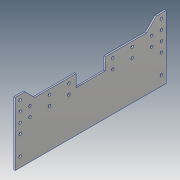
# Autodesk Inventor part: 200-40-BOGIE-CONNECTOR-06
Saved by Autodesk Inventor 2018.2 (Build 222227000, 227)
## iProperties
Manager: feesmrt
Company: FRANCOR
Part Number: 200-40-BOGIE-CONNECTOR-06
Project: Rescue Robot
Cost Center: -
Material: Aluminium 6061
Document SubType Name: Modeling
Designer: feesmrt
Engineer: feesmrt
Authority: feesmrt
Density: 2.7 g/cm^3
Appearance: Aluminium - flach
Description: Bogie Connector Verstärkungsplatte
Stock Number: 200-40-BOGIE-CONNECTOR-06
Mass: 165.052 g
Surface Area: 105.648 cm^2
Volume: 20.6315 cm^3
Subject: Rescue Robot
Author: feesmrt
Revision Number: 1
Title: Bogie Connector Verstärkungsplatte
Autodesk Inventor part; units mm, degrees
ref_plane "YZ Plane" through (0, 0, 0) normal (1, 0, 0) x (0, 1, 0)
ref_plane "XZ Plane" through (0, 0, 0) normal (0, 1, 0) x (-1, 0, 0)
ref_plane "XY Plane" through (0, 0, 0) normal (0, 0, 1) x (1, 0, 0)
sketch "Skizze1" plane through (0, 0, 0) normal (1, 0, 0) x (0, 1, 0)
  line L0 (-155, -65) -> (155, -65)
  line L1 (155, -65) -> (155, 65)
  line L2 (155, 65) -> (-155, 65)
  line L3 (-155, 65) -> (-155, -65)
  line L4 (-155, -65) -> (155, 65) construction
  line L5 (155, -65) -> (-155, 65) construction
  point P0 (0, 0)
  dimension "d43" = 310
  dimension "d44" = 130
  constraints: 12 end point, 2 midpoint, 2 parallel, 1 horizontal, 1 perpendicular
  measures "d43" distance of L1.end L2.end
  measures "d44" distance of L0.end L1.end
extrude "Grundlörper" add sketch "Skizze1" along normal blind 3
sketch "Skizze5" plane through (3, 0, 0) normal (1, 0, 0) x (0, 0, -1)
  line L0 (-65, -155) -> (65, -155) construction
  line L1 (-65, 155) -> (-65, -155) construction
  line L2 (65, 155) -> (-65, 155) construction
  line L3 (-147, 0) -> (147, 0) construction
  line L4 (0, -217) -> (0, 217) construction
  line L5 (-65, -135) -> (-45, -115)
  line L6 (-45, -115) -> (-45, -30)
  line L7 (-45, -30) -> (-20, -30)
  line L8 (-20, -30) -> (-20, 30)
  line L9 (-20, 30) -> (-45, 30)
  line L10 (-45, 30) -> (-45, 115)
  line L11 (-45, 115) -> (-65, 135)
  line L12 (-65, -135) -> (-65, 135)
  point P0 (0, 0)
  dimension "d47" = 20
  dimension "d48" = 20
  dimension "d49" = 20
  dimension "d50" = 60
  dimension "d51" = 25
  constraints: 16 end point, 3 perpendicular, 3 vertical, 2 point on line, 3 other
  measures "d47" distance from line of L0 L5.start
  measures "d48" horizontal distance of L5.start L5.end
  measures "d49" distance between parallel lines of L1 L6
  measures "d50" distance between parallel lines of L9 L7
  measures "d51" distance of L6.end L7.end
extrude "Aussschnitt" cut sketch "Skizze5" against normal through all
sketch "Skizze6" plane through (3, 0, 0) normal (1, 0, 0) x (0, 0, -1)
  line L0 (-65, -155) -> (65, -155) construction
  line L1 (-65, -135) -> (-65, -155) construction
  line L2 (-65, -145) -> (65, -145) construction
  line L3 (65, -155) -> (65, 155) construction
  line L4 (-35, -30) -> (-35, -155) construction
  line L5 (-45, -30) -> (-45, -115) construction
  line L6 (-15, 0) -> (-15, -155) construction
  line L7 (-147, 0) -> (147, 0) projected
  point P0 (-55, -145)
  point P1 (-35, -125)
  point P2 (-35, -85)
  point P3 (-35, -45)
  point P4 (-15, -125)
  point P5 (-15, -85)
  point P6 (-15, -45)
  point P7 (-35, -145)
  point P8 (-15, -145)
  point P9 (5, -145)
  point P10 (-55, 145)
  point P11 (-35, 125)
  point P12 (-35, 85)
  point P13 (-35, 45)
  point P14 (-15, 125)
  point P15 (-15, 85)
  point P16 (-15, 45)
  point P17 (-35, 145)
  point P18 (-15, 145)
  point P19 (5, -145)
  point P20 (45, -145)
  point P21 (5, 145)
  point P22 (45, 145)
  dimension "d54" = 10
  dimension "d62" = 10
  dimension "d63" = 30
  dimension "d71" = 20
  dimension "d74" = 40
  dimension "d77" = 20
  dimension "d82" = 20
  dimension "d99" = 40
  constraints: 11 symmetric about line, 9 point on line, 6 end point, 3 vertical, 2 horizontal, 1 coincident, 1 midpoint, 5 other
  measures "d54" distance from line of L1 point (-55, -145)
  measures "d62" distance between parallel lines of L5 L4
  measures "d63" distance from line of L0 point (-35, -125)
  measures "d71" distance between parallel lines of L4 L6
  measures "d74" distance of point (-35, -125) point (-35, -85)
  measures "d77" distance of point (-35, -125) point (-15, -125)
  measures "d82" distance of point (-15, -145) point (5, -145)
  measures "d99" distance of point (5, -145) point (45, -145)
hole "M5_Bohrung" at (3, -145, 55) at (3, -125, 35) at (3, -85, 35) at (3, -45, 35) at (3, -125, 15) at (3, -85, 15) at (3, -45, 15) at (3, -145, 35) at (3, -145, 15) at (3, -145, -5) at (3, 45, 35) at (3, 45, 15) at (3, 85, 35) at (3, 85, 15) at (3, 125, 35) at (3, 125, 15) at (3, 145, 55) at (3, 145, 35) at (3, 145, 15) at (3, 145, -5) at (3, 145, -45) at (3, -145, -45) direction (-1, 0, 0) diameter 5.5 end through all
